Autodesk Fusion 360 part; units mm, degrees
(part 4 of 4)
sketch "草图63" plane through (0, -12, 0) normal (0, -1, 0) x (1, 0, 0)
  arc A0 (23.0951, -99.619) -> (20.0951, -102.619) centre (23.0951, -102.619) ccw
  line L0 (20.0951, -102.619) -> (20.0951, -106.619)
  arc A1 (20.0951, -106.619) -> (23.0951, -109.619) centre (23.0951, -106.619) ccw
  line L1 (23.0951, -109.619) -> (295.896, -109.619)
  arc A2 (295.896, -109.619) -> (298.896, -106.619) centre (295.896, -106.619) ccw
  line L2 (298.896, -106.619) -> (298.896, -102.619)
  arc A3 (298.896, -102.619) -> (295.896, -99.619) centre (295.896, -102.619) ccw
  line L3 (295.896, -99.619) -> (23.0951, -99.619)
  circle A4 centre (210.895, -106.12) radius 1.1
  circle A5 centre (109.895, -106.12) radius 1.1
component "鸟" placed x (1, 0, 0) y (0, 1, 0) z (0, 0, 1) at (0, 0, 0)
hidden bodies 4
named bodies: "钢板定位板", "底壳", "pcb定位板", "PCB定位板"
